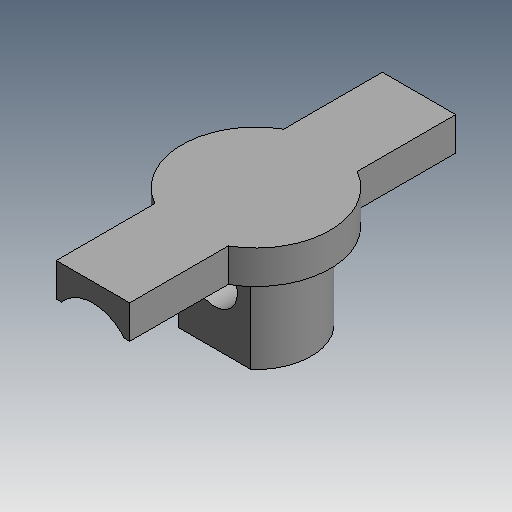
# Autodesk Inventor part: HDJSN8-45__j
Saved by Autodesk Inventor 2020 (Build 240168000, 168)
## iProperties
Part Number: HDJSN8-45__j
Material: 一般
Catalog Web Link: www.cadenas.de
Description: HDJFSN_joint-Double Joint
Vendor: MISUMI
Document SubType Name: Modeling
Designer: partserver
Manufacturer: MISUMI
Mass: 3.51425 g
Surface Area: 23.5342 cm^2
Volume: 3.51425 cm^3
Density: 1 g/cm^3
Appearance: PSOLRGB-192-192-192
Category: PARTsolutions
Company: MISUMI
PSOL_IDENT_0: {$CADENAS_DATA\23d-libs\misumi\metric\38_al_extrusions_blackets\blind\hdjfsn.prj},170 {VTYP=3D},{NB=
PSOL_IDENT_1: HDJSN8-45__j},{LINA=HDJSN8-45_},{NN=HDJFSN_joint},{DATE=08.06.2021 08:27:16},{GEOMDATE=18.09.2018 04
PSOL_IDENT_2: :29:15},{VERSION=},{LINEID=40},{WBVAR=TS},{WBNUMERIC=}  {NB=HDJSN8-45__j},{LINA=HDJSN8-45_},{KT=DUMM
PSOL_IDENT_3: Y},{PN=HDJSN8-45_},{TS=HDJSN},{TSALG=  'HDJSN' , 'Pre-Assembly Double Joint Kit' , 'HDJFSN' , 'Pre-a
PSOL_IDENT_4: ssembly Double Joint Single Item' },{MAT=316 Stainless Steel or Equivalent/Sintering},{NO=8-45},{L=4
PSOL_IDENT_5: 4},{A=9.9},{B=16},{E=11.2},{T=4.5},{S=8.0},{N=6.2},{M=6},{R=5.50},{DD=14.9},{D=20.0},{SCB=6},{SCBL=3
PSOL_IDENT_6: 5},{NON=8},{NON1=8},{MATNUT=316 Stainless Steel (or Equivalent)},{JAV=HDJSFN_},{X=5.100}
NB: HDJSN8-45__j
NN: HDJFSN_joint
NT: Double Joint
NBSYN: $PN._j
LINA: HDJSN8-45_
CATALOG: Misumi
PN: HDJSN8-45_
TS: Pre-Assembly Double Joint Kit
MAT: 316 Stainless Steel or Equivalent/Sintering
NO: 8-45
L: 44
A: 9.9
B: 16
E: 11.2
T: 4.5
S: 8
N: 6.2
R: 5.5
DD: 14.9
D: 20
SUPPLIER: MISUMI
ARTICLENO: HDJSN8-45__j
BOMINFO: HDJSN8-45_
CREATOR: CADENAS GmbH
d8: 0.000 mm
Title: HDJSN8-45_
Author: Cadenas PARTsolutions
Comments: Double Joint
Autodesk Inventor part; units mm, degrees
sketch "Sketch_1" plane through (0, 0, 0) normal (0, 0, 1) x (1, 0, 0)
  arc A0 (-4.95, 8.6889) -> (-4.95, -8.6889) centre (0, 0) ccw
  line L0 (-4.95, -8.6889) -> (-4.95, -22)
  line L1 (-4.95, -22) -> (4.95, -22)
  line L2 (4.95, -22) -> (4.95, -8.6889)
  arc A1 (4.95, -8.6889) -> (4.95, 8.6889) centre (0, 0) ccw
  line L3 (4.95, 8.6889) -> (4.95, 22)
  line L4 (4.95, 22) -> (-4.95, 22)
  line L5 (-4.95, 22) -> (-4.95, 8.6889)
  constraints: 12 end point, 4 point on circle, 2 centre point
extrude "Extrusion1" add sketch "Sketch_1" along normal blind 4.5
sketch "Sketch_2" plane through (0, 0, 0) normal (0, 1, 0) x (-1, 0, 0)
  circle A0 centre (0, 8) radius 5.5
  constraints: 1 centre point
extrude "Extrusion2" cut sketch "Sketch_2" along normal mid plane 44
sketch "Sketch_3" plane through (0, 0, 0) normal (0, 0, 1) x (1, 0, 0)
  arc A0 (-4.9135, 5.6) -> (-4.9135, -5.6) centre (0, 0) ccw
  line L0 (-4.9135, -5.6) -> (4.9135, -5.6)
  arc A1 (4.9135, -5.6) -> (4.9135, 5.6) centre (0, 0) ccw
  line L1 (4.9135, 5.6) -> (-4.9135, 5.6)
  constraints: 4 end point, 4 point on circle, 2 centre point
extrude "Extrusion3" add sketch "Sketch_3" along normal blind 16
sketch "Sketch_4" plane through (0, 0, 0) normal (0, 1, 0) x (-1, 0, 0)
  circle A0 centre (0, 8) radius 3.1
  constraints: 1 centre point
extrude "Extrusion4" cut sketch "Sketch_4" along normal mid plane 11.2
ref_plane "screw_XY" through (0, 5.6, 8) normal (0, 1, 0) x (1, 0, 0)
ref_plane "screw_YZ" through (0, 5.6, 8) normal (1, 0, 0) x (0, 0, -1)
ref_plane "screw_ZX" through (0, 5.6, 8) normal (0, 0, -1) x (0, 1, 0)
body "Solid1"
